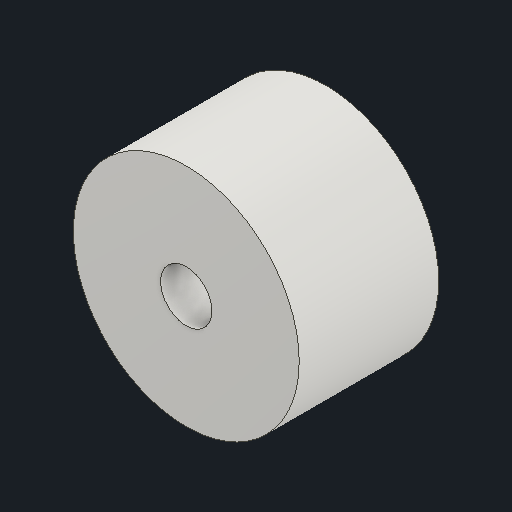
# Autodesk Inventor part: Flat Pulley2
Saved by Autodesk Inventor 2024.2 (Build 282272000, 272)
## iProperties
CustomPartVersion: 1
Created: 2024-03-22
Part Number: Flat Pulley2
Material: Steel
Document SubType Name: Modeling
Designer: LightStore
Density: 7.85 g/cm^3
Appearance: Steel
d3: 0.000 mm
d4: 0.000 mm
Author: LightStore
Autodesk Inventor part; units mm, degrees
ref_plane "YZ Plane" through (0, 0, 0) normal (1, 0, 0) x (0, 1, 0)
ref_plane "XZ Plane" through (0, 0, 0) normal (0, 1, 0) x (-1, 0, 0)
ref_plane "XY Plane" through (0, 0, 0) normal (0, 0, 1) x (1, 0, 0)
sketch "Sketch3" plane through (0, 0, 0) normal (0, 0, 1) x (1, 0, 0)
  circle A0 centre (0, 0) radius 11
  circle A1 centre (0, 0) radius 2.5
  dimension "d8" = 22
  dimension "d9" = 5
  constraints: 2 centre point, 2 coincident
  measures "d8" diameter of A0
  measures "d9" diameter of A1
extrude "Extrusion3" add sketch "Sketch3" along normal blind 5 and the other way blind 8.586
equation "\"da_D\" = 22"
equation "\"da_B\" = 15.3"
body "Solid2"
